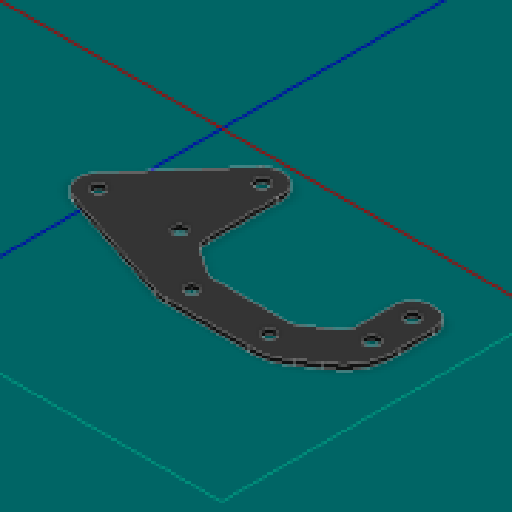
# Autodesk Inventor part: funnel_gusset_full
Saved by Autodesk Inventor 2025 (Build 290162000, 162)
## iProperties
Created: 2024-08-12
Part Number: funnel_gusset_full
Material: Acetal Resin, Black
Document SubType Name: Modeling
Designer: averey
Density: 1.425 g/cm^3
Appearance: Smooth - Black
Author: averey
Autodesk Inventor part; units mm, degrees
ref_plane "YZ Plane" through (0, 0, 0) normal (1, 0, 0) x (0, 1, 0)
ref_plane "XZ Plane" through (0, 0, 0) normal (0, 1, 0) x (-1, 0, 0)
ref_plane "XY Plane" through (0, 0, 0) normal (0, 0, 1) x (1, 0, 0)
sketch "Sketch1" plane through (0, 0, 0) normal (0, 1, 0) x (-1, 0, 0)
  circle A0 centre (-40.7913, 50.1867) radius 2.1
  circle A1 centre (-65.133, 50.1867) radius 2.1
  line L0 (-65.3307, 56.5367) -> (-38.9924, 56.5367)
  spline S0 degree 3 poles (-76.2574, 53.0916) (-75.8034, 53.4094) (-74.4464, 54.3628) (-71.9795, 55.7143) (-68.6599, 56.5178) (-66.439, 56.5367) (-65.3307, 56.5367) knots 0 0 0 0 0.147326 0.441978 0.73663 1.031282 1.031282 1.031282 1.031282
  spline S1 degree 3 poles (-89.4746, 33.9199) (-89.4746, 34.7907) (-89.485, 37.3864) (-88.662, 41.8159) (-85.6065, 46.4828) (-82.7779, 48.5258) (-81.3513, 49.5248) knots 0 0 0 0 0.176446 0.529337 0.882228 1.235119 1.235119 1.235119 1.235119
  line L1 (-81.3513, 49.5248) -> (-76.2574, 53.0916)
  line L2 (-89.4746, 23.1867) -> (-89.4746, 33.9199)
  spline S2 degree 3 poles (-83.1246, 16.8367) (-83.5996, 16.8367) (-84.5396, 16.8415) (-85.939, 17.1545) (-87.2739, 17.9007) (-88.4105, 19.0375) (-89.1576, 20.3727) (-89.4699, 21.7718) (-89.4746, 22.7117) (-89.4746, 23.1867) knots 0 0 0 0 0.123366 0.246731 0.370097 0.493463 0.616828 0.740194 0.86356 0.86356 0.86356 0.86356
  spline S3 degree 3 poles (-76.7746, 23.1867) (-76.7746, 22.7117) (-76.7794, 21.7718) (-77.0925, 20.3724) (-77.8386, 19.0375) (-78.9754, 17.9008) (-80.3107, 17.1538) (-81.7098, 16.8415) (-82.6497, 16.8367) (-83.1246, 16.8367) knots 0 0 0 0 0.123366 0.246731 0.370097 0.493463 0.616828 0.740194 0.86356 0.86356 0.86356 0.86356
  circle A2 centre (-83.1246, 23.1867) radius 2.3114
  circle A3 centre (-83.1246, 35.8867) radius 2.3114
  spline S4 degree 3 poles (-74.0669, 38.4483) (-74.5424, 38.1153) (-75.4851, 37.433) (-76.5038, 35.8783) (-76.7782, 34.4018) (-76.7746, 33.537) (-76.7746, 33.2467) knots 0 0 0 0 0.11763 0.235261 0.352891 0.411706 0.411706 0.411706 0.411706
  line L3 (-76.7746, 33.2467) -> (-76.7746, 23.1867)
  line L4 (-68.0115, 42.6883) -> (-74.0669, 38.4483)
  spline S5 degree 3 poles (-64.3693, 43.8367) (-64.7387, 43.8367) (-65.4747, 43.8285) (-66.7721, 43.5188) (-67.5576, 43.0062) (-68.0115, 42.6883) knots 0 0 0 0 0.098217 0.196435 0.343761 0.343761 0.343761 0.343761
  line L5 (-41.555, 43.8367) -> (-64.3693, 43.8367)
  spline S6 degree 3 poles (-37.9128, 42.6883) (-38.2154, 42.9002) (-38.823, 43.3156) (-40.0634, 43.806) (-41.0009, 43.8367) (-41.555, 43.8367) knots 0 0 0 0 0.098217 0.196435 0.343761 0.343761 0.343761 0.343761
  line L6 (-31.8574, 38.4483) -> (-37.9128, 42.6883)
  line L7 (-29.1496, 10.4867) -> (-29.1496, 33.2467)
  spline S7 degree 3 poles (-29.1496, 33.2467) (-29.1496, 33.8272) (-29.1679, 34.9915) (-29.8568, 36.7161) (-30.9093, 37.7887) (-31.6197, 38.2818) (-31.8574, 38.4483) knots 0 0 0 0 0.11763 0.235261 0.352891 0.411706 0.411706 0.411706 0.411706
  line L8 (-35.0553, 55.911) -> (3.1371, 43.4575)
  arc A4 (-35.0553, 55.911) -> (-38.9924, 56.5367) centre (-38.9924, 43.8367) ccw
  circle A5 centre (90.9711, -52.3822) radius 2.1844
  circle A6 centre (-22.7996, 35.8867) radius 2.1844
  circle A7 centre (1.1686, 37.4204) radius 2.0955
  arc A8 (5.9122, 33.199) -> (3.1371, 43.4575) centre (1.1686, 37.4204) ccw
  circle A9 centre (-22.7996, 10.4867) radius 2.1971 projected
  arc A10 (-29.1496, 10.4867) -> (-18.056, 6.2653) centre (-22.7996, 10.4867) ccw
  line L9 (-18.056, 6.2653) -> (5.9122, 33.199)
  point P0 (0, 0)
  point P1 (99.9514, -43.4019)
  point P2 (97.0418, -61.7217)
  dimension "d8" = 12.7
  dimension "d9" = 12.7
  constraints: 20 end point, 10 centre point, 6 point on circle, 5 tangent, 2 coincident, 1 horizontal, 1 vertical, 29 other
  measures "d8" diameter of A8
  measures "d9" diameter of A10
extrude "Extrusion1" add sketch "Sketch1" along normal blind 1.5875 contours L0 A4 L8 A8 L9 A10 L7 S7 L6 S6 L5 S5 L4 S4 L3 S3 S2 L2 S1 L1 S0
body "Solid1"
